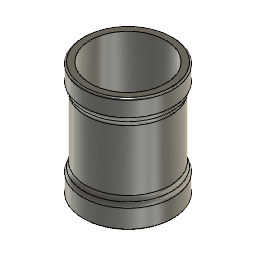
15) PLA Flexure Housing Column (Autodesk Fusion 360 design; units mm, degrees)
Autodesk Fusion 360 part; units mm, degrees
note: some values were not read from the file. Chosen so that the rebuilt part matches the saved one: which pieces of a blend or face edit are solid.
sketch "Sketch1" plane through (0, 0, 0) normal (0, 0, 1) x (1, 0, 0)
  circle A0 centre (0, 0) radius 25
  circle A1 centre (0, 0) radius 29.95
  dimension "d1" = 50
  dimension "d2" = 59.9
  constraint coincident A0.centre A1.centre
  constraint concentric A0 A1
  measures "d1" diameter of A0
  measures "d2" diameter of A1
extrude "Extrude1" add sketch "Sketch1" along normal blind 15
sketch "Sketch2" plane through (0, 0, 15) normal (0, 0, 1) x (-1, 0, 0)
  circle A0 centre (0, 0) radius 25
  circle A1 centre (0, 0) radius 29.95
  circle A2 centre (0, 0) radius 25
  circle A3 centre (0, 0) radius 28
  dimension "d5" = 50
  dimension "d6" = 56
  constraint coincident A0.centre A1.centre
  measures "d5" diameter of A2
  measures "d6" diameter of A3
extrude "Extrude2" add sketch "Sketch2" along normal blind 46.25 contours A3
sketch "Sketch3" plane through (0, 0, 61.25) normal (0, 0, 1) x (-1, 0, 0)
  circle A0 centre (0, 0) radius 25
  circle A1 centre (0, 0) radius 28
  circle A2 centre (0, 0) radius 25
  circle A3 centre (0, 0) radius 29.95
extrude "Extrude3" add sketch "Sketch3" along normal blind 15 contours A1 | A3
fillet "Fillet1" radius 5 2 faces at (-29.0842, 2.879, 61.25) (29.0842, -2.879, 15)
fillet "Fillet2" radius 1 2 edges at (27.9232, 10.8304, 76.25) (-27.9232, -10.8304, 0)
named bodies: "Flexure Housing Column"
